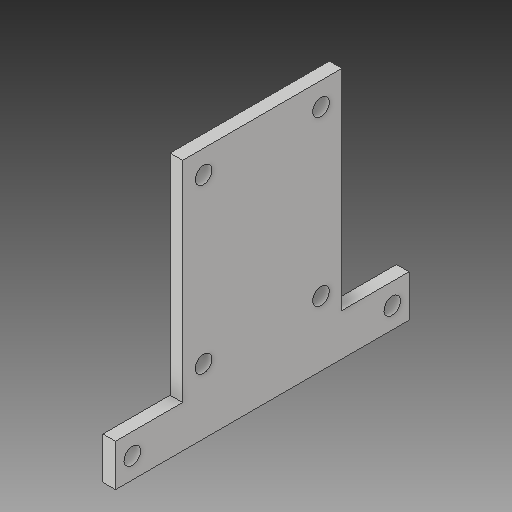
# Autodesk Inventor part: КВ33.044.704 - Панель установки принимающей платы оси Y
Saved by Autodesk Inventor 2019 (Build 230136000, 136)
## iProperties
Created: 2019-09-14
Part Number: КВ33.044.704 - Панель установки принимающей платы оси Y
Material: Типовые
Document SubType Name: Modeling
Designer: Петров Иван
Density: 1 g/cm^3
Appearance: По умолчанию
Mass: 7.57381 g
Surface Area: 60.554 cm^2
Volume: 7.57381 cm^3
Author: Петров Иван
Autodesk Inventor part; units mm, degrees
ref_plane "YZ Plane" through (0, 0, 0) normal (1, 0, 0) x (0, 1, 0)
ref_plane "XZ Plane" through (0, 0, 0) normal (0, 1, 0) x (-1, 0, 0)
ref_plane "XY Plane" through (0, 0, 0) normal (0, 0, 1) x (1, 0, 0)
sketch "Эскиз1" plane through (0, 0, 0) normal (1, 0, 0) x (0, 1, 0)
  line L0 (0, 0) -> (0, 31)
  line L1 (0, 0) -> (0, -31)
  circle A0 centre (0, 31) radius 2
  circle A1 centre (0, -31) radius 2
  line L2 (-5, 35) -> (5, 35)
  line L3 (5, 35) -> (5, -35)
  line L4 (5, -35) -> (-5, -35)
  line L5 (-5, -35) -> (-5, 35)
  line L6 (-5, 35) -> (5, -35) construction
  line L7 (5, 35) -> (-5, -35) construction
  dimension "d0" = 31
  dimension "d1" = 31
  dimension "d2" = 4
  dimension "d3" = 4
  dimension "d4" = 10
  dimension "d5" = 70
  constraints: 16 end point, 2 centre point, 2 coincident, 2 midpoint, 2 parallel, 2 vertical, 1 horizontal, 1 perpendicular
  measures "d0" distance of L0.start L0.end
  measures "d1" distance of L0.start L1.end
  measures "d2" diameter of A0
  measures "d3" diameter of A1
  measures "d4" distance of L3.end L4.end
  measures "d5" distance of L2.end L3.end
extrude "Выдавливание1" add sketch "Эскиз1" along normal blind 3
sketch "Эскиз2" plane through (3, 0, 0) normal (1, 0, 0) x (0, 0, -1)
  line L0 (35, 5) -> (-35, 5) projected
  line L1 (0, 5) -> (-14, 5)
  line L2 (-14, 5) -> (14, 5)
  line L3 (-14, 5) -> (-14, 10.5)
  line L4 (-14, 5) -> (-19, 5)
  line L5 (-19, 5) -> (19, 5)
  line L6 (19, 5) -> (19, 55)
  line L7 (19, 55) -> (-19, 55)
  line L8 (-19, 55) -> (-19, 5)
  circle A0 centre (-14, 10.5) radius 2
  line L9 (19, 30) -> (-19, 30)
  line L10 (0, 30) -> (0, 26.3042)
  circle A1 centre (14, 10.5) radius 2
  circle A2 centre (-14, 49.5) radius 2
  circle A3 centre (14, 49.5) radius 2
  point P0 (0, 0)
  dimension "d8" = 14
  dimension "d9" = 28
  dimension "d10" = 5.5
  dimension "d11" = 5
  dimension "d12" = 38
  dimension "d13" = 50
  dimension "d14" = 4
  constraints: 20 end point, 4 centre point, 4 midpoint, 3 point on line, 3 symmetric about line, 2 parallel, 2 perpendicular, 1 coincident, 1 horizontal, 1 vertical, 3 other
  measures "d8" distance of L1.start L1.end
  measures "d9" distance of L1.end L2.end
  measures "d10" distance of L1.end L3.end
  measures "d11" distance of L1.end L4.end
  measures "d12" distance of L7.end L6.end
  measures "d13" distance of L6.end L5.end
  measures "d14" diameter of A0
extrude "Выдавливание2" add sketch "Эскиз2" against normal blind 3
equation "\"d1\" = d0"
